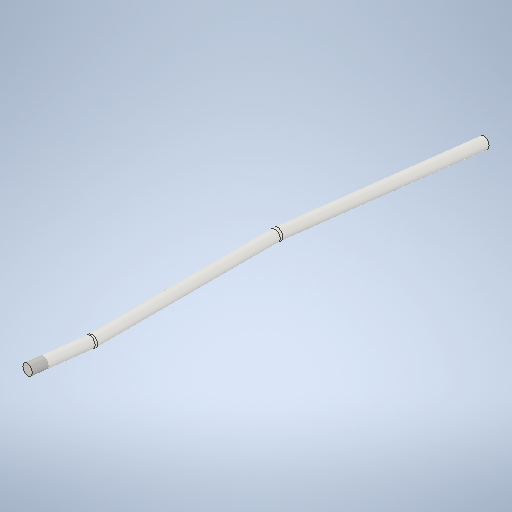
# Autodesk Inventor part: 32 - Eccentric Disk Rod
Saved by Autodesk Inventor 2025.2 (Build 292293000, 293)
## iProperties
Created: 2025-07-30
Part Number: 32 - Eccentric Disk Rod
Material: Steel AISI 1020 107 HR
Document SubType Name: Modeling
Designer: bless
Density: 7.87 g/cm^3
Appearance: Steel
Author: bless
Autodesk Inventor part; units mm, degrees
note: some values were not read from the file. Chosen so that the rebuilt part matches the saved one: bend side of "Bend Part2".
ref_plane "XZ Plane" through (0, 0, 0) normal (0, 1, 0) x (-1, 0, 0)
ref_plane "XY Plane" through (0, 0, 0) normal (0, 0, 1) x (1, 0, 0)
sketch "Sketch1" plane through (0, 0, 0) normal (0, 0, 1) x (1, 0, 0)
  circle A0 centre (0, 0) radius 1.5
  dimension "d0" = 3
  constraints: 1 centre point, 1 coincident
  measures "d0" diameter of A0
extrude "Extrusion1" add sketch "Sketch1" against normal blind 117
ref_plane "Work Plane1" through (1.5, 0, 0) normal (1, 0, 0) x (0, 1, 0)
sketch "Sketch2" plane through (1.5, 0, 0) normal (1, 0, 0) x (0, 1, 0)
  line L0 (1.5, 0) -> (1.5, -117) projected
  line L1 (1.5, 0) -> (-1.5, 0)
  line L2 (-1.5, 0) -> (-1.5, -117) projected
  line L3 (1.5, -16) -> (-1.5, -16)
  line L4 (1.5, -66) -> (-1.5, -66)
  line L5 (-1.5, -66) -> (1.5, -66)
  point P0 (0, 0)
  dimension "d4" = 0
  dimension "d5" = 16
  dimension "d6" = 50
  dimension "d17" = 0
  dimension "d18" = 0
  dimension "d19" = 3
  dimension "d20" = 3
  constraints: 8 end point, 2 horizontal, 2 parallel, 2 point on line
  measures "d4" distance from line of L0.start L1
  measures "d5" distance between parallel lines of L1 L3
  measures "d6" distance between parallel lines of L3 L4
  measures "d17" distance from line of L3.start L0
  measures "d18" distance from line of L4.start L0
  measures "d19" distance from line of L3.end L0
  measures "d20" distance from line of L4.end L0
bend part "Bend Part1" radius 5 angle 7.5 line through (1.5, -1.5, -66) along (0, 1, 0) centre toward (1, 0, 0) moving side (0, 0, -1) both sides no
sketch "Sketch3" plane through (1.5, 0, 0) normal (1, 0, 0) x (0, 1, 0)
  line L0 (-1.5, -66) -> (1.5, -66) projected
  line L1 (1.5, -66) -> (-1.5, -66)
  line L2 (-1.5, -66) -> (-1.5, -66.8484) projected
  line L3 (2.4329, -66) -> (-2.7481, -66)
  line L4 (2.4329, -16) -> (-2.7481, -16)
  point P0 (0, 0)
  dimension "d9" = 50
  dimension "d12" = 50
  dimension "d13" = 3.9329
  dimension "d14" = 3.9329
  dimension "d15" = 1.2481
  dimension "d16" = 1.2481
  constraints: 6 end point, 2 horizontal, 1 parallel, 1 point on line
  measures "d9" distance between parallel lines of L3 L4
  measures "d12" distance between parallel lines of L0 L4
  measures "d13" distance from line of L4.start L2
  measures "d14" distance from line of L3.start L2
  measures "d15" distance from line of L4.end L2
  measures "d16" distance from line of L3.end L2
bend part "Bend Part2" radius 5 angle 7.5 line through (1.5, 2.4329, -16) along (0, -1, 0) centre toward (-1, 0, 0) moving side (0, 0, 1) both sides no
thread "Thread1" size "M3x0.5" class "6g" standard "ANSI Metric M Profile" length 4
body "Solid1"
